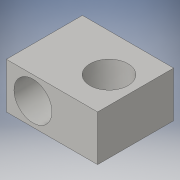
# Autodesk Inventor part: Pivot point
Saved by Autodesk Inventor 2016 (Build 200138000, 138)
## iProperties
Created: 2016-03-19
Part Number: Pivot point
Material: Generic
Document SubType Name: Modeling
Designer: matth_000
Density: 1 g/cm^3
Appearance: Default
Author: matth_000
Autodesk Inventor part; units mm, degrees
ref_plane "YZ Plane" through (0, 0, 0) normal (1, 0, 0) x (0, 1, 0)
ref_plane "XZ Plane" through (0, 0, 0) normal (0, 1, 0) x (-1, 0, 0)
ref_plane "XY Plane" through (0, 0, 0) normal (0, 0, 1) x (1, 0, 0)
sketch "Sketch1" plane through (0, 0, 0) normal (0, 1, 0) x (-1, 0, 0)
  line L0 (0, 0) -> (-30.48, 0)
  line L1 (-30.48, 0) -> (-30.48, -25.4)
  line L2 (-30.48, -25.4) -> (0, -25.4)
  line L3 (0, -25.4) -> (0, 0)
  dimension "d0" = 30.48
  dimension "d1" = 25.4
  constraints: 8 end point, 2 parallel, 1 horizontal, 1 perpendicular
  measures "d0" distance of L2.end L1.end
  measures "d1" distance of L1.end L0.end
extrude "Extrusion1" add sketch "Sketch1" along normal blind 15.24
sketch "Sketch4" plane through (30.48, 0, -25.4) normal (0, 0, -1) x (-1, 0, 0)
  circle A0 centre (21.59, 7.62) radius 6.35
  line L0 (30.48, 0) -> (30.48, 15.24) projected
  dimension "d14" = 12.7
  dimension "d15" = 8.89
  constraints: 1 centre point
  measures "d14" diameter of A0
  measures "d15" distance from line of L0 A0.centre
extrude "Extrusion4" cut sketch "Sketch4" against normal blind 25.4
sketch "Sketch5" plane through (0, 15.24, 0) normal (0, 1, 0) x (1, 0, 0)
  circle A0 centre (21.59, 12.7) radius 6.35
  line L0 (30.48, 0) -> (30.48, 25.4) projected
  point P0 (0, 0)
  dimension "d18" = 12.7
  dimension "d19" = 8.89
  constraints: 1 centre point
  measures "d18" diameter of A0
  measures "d19" distance from line of L0 A0.centre
extrude "Extrusion5" cut sketch "Sketch5" against normal blind 15.24
body "Solid1"
